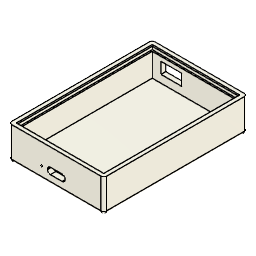
Luxmeter_Case (Autodesk Fusion 360 design; units mm, degrees)
Autodesk Fusion 360 part; units mm, degrees
sketch "Sketch1" plane through (0, 0, 0) normal (0, 0, 1) x (1, 0, 0)
  line L0 (0, 0) -> (43, 0)
  line L1 (43, 0) -> (43, 68)
  line L2 (43, 68) -> (0, 68)
  line L3 (0, 68) -> (0, 0)
  line L4 (-3, 71) -> (-3, -3)
  line L5 (-3, -3) -> (46, -3)
  line L6 (46, -3) -> (46, 71)
  line L7 (46, 71) -> (-3, 71)
  dimension "d1" = 68
  dimension "d2" = 43
  dimension "d3" = 3
  constraint horizontal L0
  constraint vertical L1
  constraint horizontal L2
  constraint vertical L3
  constraint coincident L0.start L3.end
  measures "d1" distance of L0.start L2.end
  measures "d2" distance of L0.start L0.end
extrude "Extrude1" add sketch "Sketch1" along normal blind 17
extrude "Extrude2" add sketch "Sketch1" along normal blind 3 contours L0 L1 L2 L3
sketch "Sketch2" plane through (0, 0, 17) normal (0, 0, 1) x (-1, 0, 0)
  line L0 (0, 0) -> (0, -68)
  line L1 (0, -68) -> (-43, -68)
  line L2 (-43, -68) -> (-43, 0)
  line L3 (-43, 0) -> (0, 0)
  line L4 (-46, -71) -> (3, -71)
  line L5 (3, -71) -> (3, 3)
  line L6 (3, 3) -> (-46, 3)
  line L7 (-46, 3) -> (-46, -71)
  line L8 (0.75, 0.75) -> (0.75, -68.75)
  line L9 (0.75, -68.75) -> (-43.75, -68.75)
  line L10 (-43.75, -68.75) -> (-43.75, 0.75)
  line L11 (-43.75, 0.75) -> (0.75, 0.75)
  line L12 (0, -68) -> (-43, -68)
  line L13 (-43, -68) -> (-43, 0)
  line L14 (-43, 0) -> (0, 0)
  line L15 (0, 0) -> (0, -68)
  dimension "d8" = -0.75
  dimension "d9" = 0
  measures "d9" distance of L3
extrude "Extrude3" cut sketch "Sketch2" against normal blind 2 contours L8 L9 L10 L11
sketch "Sketch3" plane through (0, 71, 0) normal (0, 1, 0) x (-1, 0, 0)
  line L0 (-46, 0) -> (3, 0)
  line L1 (3, 0) -> (3, 17)
  line L2 (3, 17) -> (-46, 17)
  line L3 (-46, 17) -> (-46, 0)
  line L4 (-15.118, 12.767) -> (-4.518, 12.767)
  line L5 (-4.518, 12.767) -> (-4.518, 6.967)
  line L6 (-4.518, 6.967) -> (-15.118, 6.967)
  line L7 (-15.118, 6.967) -> (-15.118, 12.767)
  line L8 (0, 3) -> (-43, 3)
  line L9 (-43, 3) -> (0, 3)
  dimension "d12" = 5.8
  dimension "d13" = 10.6
  dimension "d14" = 7.518
  dimension "d15" = 43
  dimension "d16" = 3.967
  constraint horizontal L4
  constraint vertical L5
  constraint horizontal L6
  constraint vertical L7
  measures "d12" distance of L4.start L6.end
  measures "d13" distance of L4.start L4.end
  measures "d14" distance of L1 L5
  measures "d15" distance of L8.start L8.end
  measures "d16" distance of L6 L9
extrude "Extrude4" cut sketch "Sketch3" against normal blind 3 contours L4 L5 L6 L7
sketch "Sketch4" plane through (0, -3, 0) normal (0, -1, 0) x (1, 0, 0)
  line L0 (-3, 0) -> (46, 0)
  line L1 (46, 0) -> (46, 17)
  line L2 (46, 17) -> (-3, 17)
  line L3 (-3, 17) -> (-3, 0)
  line L4 (16.95, 6.137) -> (16.95, 6.437)
  arc A0 (26.05, 6.437) -> (24.55, 7.937) centre (24.55, 6.437) ccw
  line L5 (24.55, 4.637) -> (18.45, 4.637)
  line L6 (26.05, 6.437) -> (26.05, 6.137)
  line L7 (18.45, 7.937) -> (24.55, 7.937)
  arc A1 (16.95, 6.137) -> (18.45, 4.637) centre (18.45, 6.137) ccw
  arc A2 (24.55, 4.637) -> (26.05, 6.137) centre (24.55, 6.137) ccw
  line L8 (24.55, 4.637) -> (18.45, 4.637)
  arc A3 (18.45, 7.937) -> (16.95, 6.437) centre (18.45, 6.437) ccw
  arc A4 (24.55, 4.637) -> (26.05, 6.137) centre (24.55, 6.137) ccw
  line L9 (18.45, 7.937) -> (24.55, 7.937)
  arc A5 (26.05, 6.437) -> (24.55, 7.937) centre (24.55, 6.437) ccw
  arc A6 (18.45, 7.937) -> (16.95, 6.437) centre (18.45, 6.437) ccw
  line L10 (26.05, 6.437) -> (26.05, 6.137)
  line L11 (16.95, 6.137) -> (16.95, 6.437)
  arc A7 (16.95, 6.137) -> (18.45, 4.637) centre (18.45, 6.137) ccw
  line L12 (21.5, 17) -> (21.5, 0)
  circle A8 centre (13.95, 6.287) radius 0.5
  dimension "d19" = 0
  dimension "d37" = 1
  constraint midpoint L2 L12.start
  constraint midpoint L0 L12.end
  measures "d37" diameter of A8
extrude "Extrude5" cut sketch "Sketch4" against normal blind 3 contours A0 L5 L6 L7 A2 L8 A4 L9 A5 L10 L12 | L4 L5 L7 A1 L8 A3 L9 A6 L11 A7 L12 | A8
fillet "Fillet1" radius 0.5 4 edges at (9.818, 71, 12.767) (4.518, 71, 9.867) (15.118, 71, 9.867) (9.818, 71, 6.967)
chamfer "Chamfer1" distance 0.1 angle 45 8 edges at (25.6107, 0, 7.4977) (21.5, 0, 7.937) (17.3893, 0, 7.4977) (16.95, 0, 6.287) (17.3893, 0, 5.0763) (21.5, 0, 4.637) (25.6107, 0, 5.0763) (26.05, 0, 6.287)
chamfer "Chamfer2" distance 0.3 distance2 0.5 4 edges at (43.75, 34, 17) (21.5, -0.75, 17) (-0.75, 34, 17) (21.5, 68.75, 17) measured on face at (-2.25, 22.4167, 17) measured on face at (-2.25, 22.4167, 17) measured on face at (-2.25, 22.4167, 17) measured on face at (-2.25, 22.4167, 17)
fillet "Fillet2" radius 1.5 8 edges at (46, 71, 8.5) (-3, 71, 8.5) (-3, -3, 8.5) (46, -3, 8.5) (46, 34, 0) (21.5, 71, 0) (-3, 34, 0) (21.5, -3, 0)
sketch "Sketch6" plane through (0, 0, 0) normal (0, 0, -1) x (1, 0, 0)
  line L0 (-1.5, -69.5) -> (44.5, -69.5)
  line L1 (44.5, -69.5) -> (44.5, 1.5)
  line L2 (44.5, 1.5) -> (-1.5, 1.5)
  line L3 (-1.5, 1.5) -> (-1.5, -69.5)
  line L4 (18.5, -61.5) -> (-1.5, -61.5) construction
  line L5 (-1.5, -61.5) -> (-1.5, -69.5) construction
  line L6 (-1.5, -69.5) -> (18.5, -69.5) construction
  line L7 (18.5, -69.5) -> (18.5, -61.5) construction
  dimension "d39" = 4
  dimension "d40" = 0
  dimension "d41" = 8
  dimension "d42" = 20
  text T0 "V 1.0" font "Arial Black" height 4 align centre middle in box 20 x 8 at (18.5, -61.5) x (-1, 0) y (0, -1) spacing 1
  constraint coincident L0.start
extrude "Extrude6" cut sketch "Sketch6" against normal blind 1 text T0
equation "d40 = 'V 1.0'"
